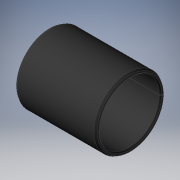
# Autodesk Inventor part: DBB1520
Saved by Autodesk Inventor 2019 (Build 230136000, 136)
## iProperties
Created: 2024-06-19
Part Number: DBB1520
Material: Generic
Catalog Web Link: www.cadenas.de
Description: DBB01-Bushing
Vendor: DAIDO
Document SubType Name: Modeling
Designer: psAdmin
Manufacturer: DAIDO
Mass: 0.99003 g
Surface Area: 21.0425 cm^2
Volume: 0.99003 cm^3
Density: 1 g/cm^3
Appearance: PSOLRGB-175-175-175
Category: PARTsolutions
Company: DAIDO
Title: DBB1520
Author: Cadenas PARTsolutions
Comments: Bushing
PSOL_IDENT_0: {$CADENAS_DATA/23d-libs/daido/resin/daibest_dbb01/bushing.prj},155 {VTYP=3D},{NB=DBB1520},{LINA=DBB1
PSOL_IDENT_1: 520},{NN=DBB01},{DATE=22.01.2019 23:13:55},{GEOMDATE=16.01.2018 02:23:26},{VERSION=},{LINEID=1380},{
PSOL_IDENT_2: WBVAR=},{WBNUMERIC=}  {NB=DBB1520},{LINA=DBB1520},{KT=DUMMY},{CNSORDERNO=DBB1520},{ID=15},{IDH=17},{
PSOL_IDENT_3: IDT=H7(+0.018/0)},{SD=15},{SDT=h7(0/-0.018)},{OD=17},{ODT=+0.073/+0.038},{T=1.0},{TT=-0.020/-0.060},
PSOL_IDENT_4: {L=20},{LT=0/-0.3}
NB: DBB1520
NN: DBB01
NT: Bushing
NBSYN: $CNSORDERNO.
LINA: DBB1520
CATALOG: DAIDO METAL
CNSORDERNO: DBB1520
ID: 15
IDH: 17
IDT: H7(+0.018/0)
SD: 15
SDT: h7(0/-0.018)
OD: 17
ODT: +0.073/+0.038
T: 1
TT: -0.020/-0.060
L: 20
LT: 0/-0.3
SUPPLIER: DAIDO
ARTICLENO: DBB1520
BOMINFO: DBB1520
CREATOR: CADENAS GmbH
Autodesk Inventor part; units mm, degrees
ref_plane "YZ Plane" through (0, 0, 0) normal (1, 0, 0) x (0, 1, 0)
ref_plane "XZ Plane" through (0, 0, 0) normal (0, 1, 0) x (-1, 0, 0)
ref_plane "XY Plane" through (0, 0, 0) normal (0, 0, 1) x (1, 0, 0)
sketch "Sketch_1" plane through (0, 0, 0) normal (0, 0, 1) x (1, 0, 0)
  line L0 (20, 0) -> (0, 0)
  line L1 (0, 7.8) -> (0.3, 7.5)
  line L2 (0.3, 7.5) -> (19.7, 7.5)
  line L3 (19.7, 7.5) -> (20, 7.8)
  line L4 (20, 7.8) -> (20, 8.2113)
  line L5 (20, 8.2113) -> (19.5, 8.5)
  line L6 (19.5, 8.5) -> (0.5, 8.5)
  line L7 (0.5, 8.5) -> (0, 8.2113)
  line L8 (0, 8.2113) -> (0, 7.8)
  constraints: 18 end point
revolve "Revolution1" add sketch "Sketch_1" angle 360 about axis through (20, 0, 0) along (1, 0, 0)
sketch "Sketch_3" plane through (0, 0, 0) normal (1, 0, 0) x (0, 1, 0)
  line L0 (0.085, -1) -> (-0.085, -1)
  line L1 (-0.085, -1) -> (-0.085, -9.5)
  line L2 (-0.085, -9.5) -> (0.085, -9.5)
  line L3 (0.085, -9.5) -> (0.085, -1)
  constraints: 8 end point
extrude "Extrusion1" cut sketch "Sketch_3" along normal blind 20
body "Solid1"
